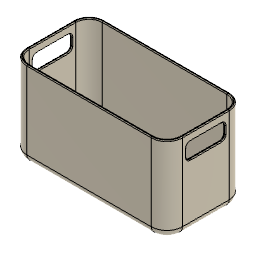
Drawer (Autodesk Fusion 360 design; units mm, degrees)
part number: 2026-06-12-13-05-57-181
Autodesk Fusion 360 part; units mm, degrees
sketch "Sketch1" plane through (0, 0, 0) normal (0, 0, 1) x (1, 0, 0)
  line L0 (-80, 50) -> (80, 50)
  line L1 (100, 30) -> (100, -30)
  line L2 (80, -50) -> (-80, -50)
  line L3 (-100, -30) -> (-100, 30)
  line L4 (-100, 50) -> (100, -50) construction
  line L5 (100, 50) -> (-100, -50) construction
  arc A0 (-80, 50) -> (-100, 30) centre (-80, 30) ccw
  arc A1 (100, 30) -> (80, 50) centre (80, 30) ccw
  arc A2 (80, -50) -> (100, -30) centre (80, -30) ccw
  arc A3 (-100, -30) -> (-80, -50) centre (-80, -30) ccw
  dimension "d1" = 200
  dimension "d2" = 100
  dimension "d5" = 20
  constraint horizontal L0
  constraint perpendicular L0 L1
  constraint parallel L0 L2
  constraint parallel L1 L3
  constraint coincident L4 origin
  constraint coincident L5 origin
  constraint coincident L4.start L3
  constraint coincident L4.start L0
  constraint tangent L3 A0
  constraint tangent L0 A0
  constraint coincident L5.start L0
  constraint coincident L5.start L1
  constraint tangent L0 A1
  constraint tangent L1 A1
  constraint equal A0 A1
  constraint coincident L4.end L1
  constraint coincident L4.end L2
  constraint tangent L1 A2
  constraint tangent L2 A2
  constraint equal A0 A2
  constraint coincident L5.end L2
  constraint coincident L5.end L3
  constraint tangent L2 A3
  constraint tangent L3 A3
  constraint equal A0 A3
  measures "d1" distance of L4.end L5.end
  measures "d2" distance of L5.start L4.end
  measures "d5" radius of A0
extrude "Extrude1" add sketch "Sketch1" along normal blind 110
sketch "Sketch2" plane through (100, 0, 0) normal (1, 0, 0) x (0, 1, 0)
  line L0 (-30, 0) -> (30, 0)
  line L1 (30, 0) -> (30, 110)
  line L2 (30, 110) -> (-30, 110)
  line L3 (-30, 110) -> (-30, 0)
  line L4 (20, 100) -> (-20, 100)
  line L5 (-25, 95) -> (-25, 85)
  line L6 (-20, 80) -> (20, 80)
  line L7 (25, 85) -> (25, 95)
  line L8 (25, 100) -> (-25, 80) construction
  line L9 (-25, 100) -> (25, 80) construction
  arc A0 (-20, 100) -> (-25, 95) centre (-20, 95) ccw
  arc A1 (25, 95) -> (20, 100) centre (20, 95) ccw
  arc A2 (20, 80) -> (25, 85) centre (20, 85) ccw
  arc A3 (-25, 85) -> (-20, 80) centre (-20, 85) ccw
  point P0 (0, 90)
  dimension "d6" = 50
  dimension "d7" = 20
  dimension "d9" = 5
  dimension "d10" = 5
  dimension "d18" = 10
  constraint horizontal L4
  constraint perpendicular L4 L5
  constraint parallel L4 L6
  constraint parallel L5 L7
  constraint coincident L8 P0
  constraint coincident L9 P0
  constraint coincident L9.start L5
  constraint coincident L9.start L4
  constraint tangent L5 A0
  constraint tangent L4 A0
  constraint coincident L8.start L4
  constraint coincident L8.start L7
  constraint tangent L4 A1
  constraint tangent L7 A1
  constraint equal A0 A1
  constraint coincident L9.end L7
  constraint coincident L9.end L6
  constraint tangent L7 A2
  constraint tangent L6 A2
  constraint equal A0 A2
  constraint coincident L8.end L6
  constraint coincident L8.end L5
  constraint tangent L6 A3
  constraint tangent L5 A3
  measures "d6" distance of L8.end L9.end
  measures "d7" distance of L9.start L8.end
  measures "d9" radius of A0
  measures "d10" radius of A3
  measures "d18" distance of L2 L4
fillet "Fillet3" radius 10 8 edges at (94.1421, -44.1421, 0) (0, -50, 0) (-94.1421, -44.1421, 0) (-100, 0, 0) (-94.1421, 44.1421, 0) (0, 50, 0) (94.1421, 44.1421, 0) (100, 0, 0)
shell "Shell1" thickness 3 removed faces 1 at (-26.6667, -16.6667, 110)
extrude "Extrude2" cut sketch "Sketch2" against normal through all contours L4 L5 L6 L7 A0 A1 A2 A3
fillet "Fillet1" radius 1 8 edges at (0, 50, 110) (-94.1421, 44.1421, 110) (-100, 0, 110) (-94.1421, -44.1421, 110) (0, -50, 110) (94.1421, -44.1421, 110) (100, 0, 110) (94.1421, 44.1421, 110)
fillet "Fillet2" radius 1 32 edges at (-100, 25, 90) (-100, 23.5355, 98.5355) (-100, 0, 100) (-100, -23.5355, 98.5355) (-100, -25, 90) (-100, -23.5355, 81.4645) (-100, 0, 80) (-100, 23.5355, 81.4645) (-97, -25, 90) (-97, -23.5355, 98.5355) (-97, 0, 100) (-97, 23.5355, 98.5355) (-97, 25, 90) (-97, 23.5355, 81.4645) (-97, 0, 80) (-97, -23.5355, 81.4645) (100, -25, 90) (100, -23.5355, 98.5355) (100, 0, 100) (100, 23.5355, 98.5355) (100, 25, 90) (100, 23.5355, 81.4645) (100, 0, 80) (100, -23.5355, 81.4645) (97, 25, 90) (97, 23.5355, 98.5355) (97, 0, 100) (97, -23.5355, 98.5355) (97, -25, 90) (97, -23.5355, 81.4645) (97, 0, 80) (97, 23.5355, 81.4645)
fillet "Fillet4" radius 1 8 edges at (-97, 0, 110) (-92.0208, 42.0208, 110) (0, 47, 110) (92.0208, 42.0208, 110) (97, 0, 110) (92.0208, -42.0208, 110) (0, -47, 110) (-92.0208, -42.0208, 110)
